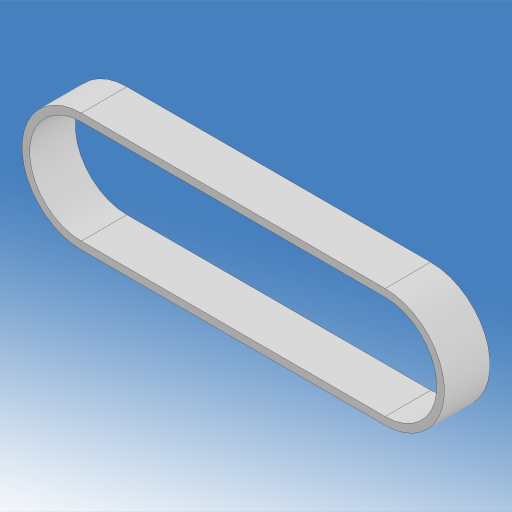
# Autodesk Inventor part: MasterSketch
Saved by Autodesk Inventor 2024 (Build 280153000, 153)
## iProperties
Created: 2024-03-21
Part Number: MasterSketch
Material: Generic
Document SubType Name: Modeling
Designer: seene
Density: 1 g/cm^3
Appearance: Default
Author: seene
Autodesk Inventor part; units mm, degrees
ref_plane "YZ Plane" through (0, 0, 0) normal (1, 0, 0) x (0, 1, 0)
ref_plane "XZ Plane" through (0, 0, 0) normal (0, 1, 0) x (-1, 0, 0)
ref_plane "XY Plane" through (0, 0, 0) normal (0, 0, 1) x (1, 0, 0)
sketch "Chassis" plane through (0, 0, 0) normal (0, 0, 1) x (1, 0, 0)
  line L0 (0, 0) -> (660.4, 0) construction
  line L1 (660.4, 0) -> (660.4, 152.4) construction
  line L2 (660.4, 152.4) -> (0, 152.4) construction
  line L3 (0, 152.4) -> (0, 0) construction
  line L4 (50.8, 127) -> (609.6, 127) construction
  line L5 (635, 101.6) -> (635, 50.8) construction
  line L6 (609.6, 25.4) -> (50.8, 25.4) construction
  line L7 (25.4, 50.8) -> (25.4, 101.6) construction
  arc A0 (50.8, 127) -> (25.4, 101.6) centre (50.8, 101.6) ccw construction
  arc A1 (25.4, 50.8) -> (50.8, 25.4) centre (50.8, 50.8) ccw construction
  arc A2 (609.6, 25.4) -> (635, 50.8) centre (609.6, 50.8) ccw construction
  arc A3 (635, 101.6) -> (609.6, 127) centre (609.6, 101.6) ccw construction
  dimension "d0" = 660.4
  dimension "d1" = 152.4
  dimension "d3" = 25.4
  dimension "d4" = 25.4
  constraints: 16 end point, 8 point on circle, 8 tangent, 4 centre point, 4 parallel, 3 equal radius, 2 perpendicular, 1 horizontal, 3 other
  measures "d0" distance of L2.end L1.end
  measures "d1" distance of L2.end L0.start
  measures "d3" distance between parallel lines of L2 L4
  measures "d4" radius of A0
sketch "Motor and motor mount" plane through (0, 0, 0) normal (0, 0, 1) x (1, 0, 0)
  line L0 (152.5322, 25.4) -> (519.6657, 25.4) construction
  line L1 (519.6657, 25.4) -> (519.6657, 127) construction
  line L2 (519.6657, 127) -> (152.5322, 127) construction
  line L3 (152.5322, 127) -> (152.5322, 25.4) construction
  line L4 (152.5322, 31.75) -> (519.6657, 31.75) construction
  line L5 (168.5983, 31.75) -> (502.5549, 31.75) construction
  line L6 (502.5549, 31.75) -> (502.5549, 131.1076) construction
  line L7 (502.5549, 131.1076) -> (168.5983, 131.1076) construction
  line L8 (168.5983, 131.1076) -> (168.5983, 31.75) construction
  circle A0 centre (459.6569, 62.4006) radius 45.974 construction
  line L9 (50.8, 127) -> (609.6, 127) construction
  line L10 (168.5983, 121.0746) -> (502.5549, 121.0746) construction
  line L11 (76.2661, 152.2106) -> (76.2661, 127) construction
  line L12 (0, 152.4) -> (0, 0) construction
  line L13 (609.6, 25.4) -> (50.8, 25.4) construction
  circle A1 centre (459.6569, 62.4006) radius 6.35 construction
  point P0 (76.2661, 139.6053)
  dimension "d5" = 367.1334
  dimension "d6" = 101.6
  dimension "d8" = 6.35
  dimension "d9" = 333.9566
  dimension "d10" = 17.1108
  dimension "d12" = 42.898
  dimension "d14" = 4.1076
  dimension "d15" = 5.9254
  dimension "d16" = 58.674
  dimension "d17" = 76.2661
  dimension "d18" = 76.2661
  dimension "d19" = 91.948
  dimension "d20" = 12.7
  constraints: 22 end point, 7 point on line, 4 horizontal, 4 parallel, 2 centre point, 2 perpendicular, 1 coincident, 1 midpoint, 1 vertical
  measures "d5" distance of L2.end L1.end
  measures "d6" distance of L1.end L0.end
  measures "d8" distance between parallel lines of L0 L4
  measures "d9" distance of L6.end L7.end
  measures "d10" distance between parallel lines of L1 L6
  measures "d12" distance from line of L6 A0.centre
  measures "d14" distance between parallel lines of L9 L7
  measures "d15" distance between parallel lines of L9 L10
  measures "d16" distance from line of A0.centre L10
  measures "d17" distance from line of point (76.266, 139.605) L12
  measures "d18" distance between parallel lines of L11 L3
  measures "d19" diameter of A0
  measures "d20" diameter of A1
sketch "Flipper drive rails" plane through (0, 0, 0) normal (0, 0, 1) x (1, 0, 0)
  circle A0 centre (584.2, 48.1766) radius 12.7 construction
  line L0 (660.4, 0) -> (660.4, 152.4) construction
  line L1 (0, 0) -> (660.4, 0) construction
  circle A1 centre (76.2, 48.1766) radius 12.7 construction
  line L2 (0, 152.4) -> (0, 0) construction
  circle A2 centre (76.2, 48.1766) radius 58.166 construction
  circle A3 centre (584.2, 48.1766) radius 58.166 construction
  circle A4 centre (459.6569, 62.4006) radius 45.974 construction
  dimension "d21" = 25.4
  dimension "d22" = 76.2
  dimension "d24" = 25.4
  dimension "d25" = 76.2
  dimension "d27" = 116.332
  dimension "d28" = 116.332
  dimension "d49" = 14.224
  constraints: 4 centre point, 2 coincident, 1 horizontal alignment
  measures "d21" diameter of A0
  measures "d22" distance from line of L0 A0.centre
  measures "d24" diameter of A1
  measures "d25" distance from line of A1.centre L2
  measures "d27" diameter of A2
  measures "d28" diameter of A3
  measures "d49" vertical distance of A0.centre A4.centre
sketch "Flipper Gears" plane through (0, 0, 0) normal (0, 0, 1) x (1, 0, 0)
  circle A0 centre (172.9676, 98.1053) radius 29.845 construction
  circle A1 centre (217.0566, 68.0834) radius 23.495 construction
  circle A2 centre (157.4388, 37.1885) radius 33.02 construction
  circle A3 centre (157.4388, 37.1885) radius 23.8125 construction
  circle A4 centre (76.2, 48.1766) radius 58.166 construction
  circle A5 centre (584.2, 48.1766) radius 12.7 construction
  circle A6 centre (584.2, 48.1766) radius 86.36 construction
  circle A7 centre (476.7097, 24.0144) radius 23.8125 construction
  circle A8 centre (476.7097, 24.0144) radius 33.02 construction
  circle A9 centre (422.0639, 55.0924) radius 29.845 construction
  circle A10 centre (385.32, 16.4266) radius 23.495 construction
  line L0 (253.1246, 92.8334) -> (396.8286, 92.8334) construction
  line L1 (396.8286, 92.8334) -> (396.8286, 43.3334) construction
  line L2 (396.8286, 43.3334) -> (253.1246, 43.3334) construction
  line L3 (253.1246, 43.3334) -> (253.1246, 92.8334) construction
  line L4 (349.252, 16.4266) -> (385.32, 16.4266) construction
  line L5 (217.0566, 68.0834) -> (253.1246, 68.0834) construction
  line L6 (205.548, 41.1766) -> (349.252, 41.1766) construction
  line L7 (349.252, 41.1766) -> (349.252, -8.3234) construction
  line L8 (349.252, -8.3234) -> (205.548, -8.3234) construction
  line L9 (205.548, -8.3234) -> (205.548, 41.1766) construction
  circle A11 centre (76.2, 48.1766) radius 86.36 construction
  line L10 (76.2, 48.1766) -> (584.2, 48.1766) construction
  line L11 (76.2, -50.8834) -> (584.2, -50.8834) construction
  line L12 (584.2, 147.2366) -> (76.2, 147.2366) construction
  arc A12 (76.2, 147.2366) -> (76.2, -50.8834) centre (76.2, 48.1766) ccw construction
  arc A13 (584.2, -50.8834) -> (584.2, 147.2366) centre (584.2, 48.1766) ccw construction
  circle A14 centre (76.2, 48.1766) radius 99.06 construction
  line L13 (76.2, 48.1766) -> (584.2, 48.1766) construction
  line L14 (76.2, -38.1834) -> (584.2, -38.1834) construction
  line L15 (584.2, 134.5366) -> (76.2, 134.5366) construction
  arc A15 (76.2, 134.5366) -> (76.2, -38.1834) centre (76.2, 48.1766) ccw construction
  arc A16 (584.2, -38.1834) -> (584.2, 134.5366) centre (584.2, 48.1766) ccw construction
  point P0 (0, 0)
  point P1 (330.2, 48.1766)
  point P2 (330.2, 48.1766)
  dimension "d29" = 59.69
  dimension "d30" = 46.99
  dimension "d31" = 66.04
  dimension "d32" = 47.625
  dimension "d34" = 172.72
  dimension "d35" = 47.625
  dimension "d36" = 66.04
  dimension "d37" = 59.69
  dimension "d38" = 46.99
  dimension "d39" = 143.704
  dimension "d40" = 49.5
  dimension "d43" = 36.068
  dimension "d48" = 24.1623
  dimension "d50" = 31.75
  dimension "d51" = 38.6658
  dimension "d52" = 143.704
  dimension "d53" = 49.5
  dimension "d54" = 36.068
  dimension "d55" = 51.6568
  dimension "d60" = 172.72
  dimension "d62" = 12.7
  constraints: 36 end point, 15 centre point, 15 tangent, 8 point on circle, 6 horizontal, 5 parallel, 4 coincident, 4 midpoint, 2 perpendicular, 1 concentric, 1 vertical
  measures "d29" diameter of A0
  measures "d30" diameter of A1
  measures "d31" diameter of A2
  measures "d32" diameter of A3
  measures "d34" diameter of A6
  measures "d35" diameter of A7
  measures "d36" diameter of A8
  measures "d37" diameter of A9
  measures "d38" diameter of A10
  measures "d39" distance of L0.start L0.end
  measures "d40" distance of L2.end L0.start
  measures "d43" distance from line of L3 L5.start
  measures "d48" vertical distance of A5.centre A7.centre
  measures "d50" vertical distance of A5.centre L4.end
  measures "d51" vertical distance of A9.centre L4.end
  measures "d52" distance of L7.end L8.end
  measures "d53" distance between parallel lines of L8 L6
  measures "d54" distance from line of L4.end L7
  measures "d55" distance between parallel lines of L6 L0
  measures "d60" diameter of A11
  measures "d62" radial gap between concentric circles of A11 A14
sketch "Flipper" plane through (0, 0, 0) normal (0, 0, 1) x (1, 0, 0)
  circle A0 centre (76.2, 48.1766) radius 63.5 construction
  circle A1 centre (-169.7482, 3.0916) radius 41.275 construction
  circle A2 centre (76.2, 48.1766) radius 86.36 construction
  line L0 (-169.7482, -38.1834) -> (76.2, -38.1834) construction
  point P0 (0, 0)
  point P1 (584.2, 48.1766)
  dimension "d57" = 82.55
  dimension "d58" = 172.72
  dimension "d56" = 127
  dimension "d59" = 245.9482
  constraints: 3 horizontal, 2 coincident, 2 end point, 2 vertical alignment, 1 centre point, 4 other
  measures "d56" diameter of A0
  measures "d59" horizontal distance of point (76.2, 48.177) point (-169.748, 3.092)
sketch "Sketch6" plane through (0, 0, 0) normal (0, 0, 1) x (1, 0, 0)
  line L0 (584.2, 147.2366) -> (76.2, 147.2366) projected
  arc A0 (76.2, 147.2366) -> (76.2, -50.8834) centre (76.2, 48.1766) ccw projected
  line L1 (584.2, 134.5366) -> (76.2, 134.5366) projected
  circle A1 centre (76.2, 48.1766) radius 86.36 projected
  line L2 (76.2, -38.1834) -> (584.2, -38.1834) projected
  line L3 (76.2, -50.8834) -> (584.2, -50.8834) projected
  arc A2 (584.2, -50.8834) -> (584.2, 147.2366) centre (584.2, 48.1766) ccw projected
  circle A3 centre (584.2, 48.1766) radius 86.36 projected
  point P0 (0, 0)
extrude "Extrusion1" add sketch "Sketch6" along normal blind 76.2
body "Solid1"
